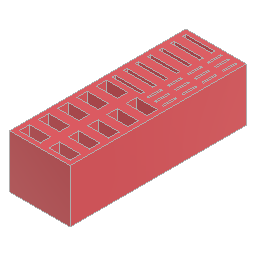
Digital-Storage-Carrier (Autodesk Fusion 360 design; units mm, degrees)
Autodesk Fusion 360 part; units mm, degrees
sketch "Sketch1 (1)" plane through (0, 0, 0) normal (0, 0, 1) x (1, 0, 0)
  line L0 (0, -297.942, 53.175) -> (51.1, -297.942, 53.175)
  line L1 (51.1, -297.942, 53.175) -> (51.1, -148.972, 53.175)
  line L2 (51.1, -148.972, 53.175) -> (0, -148.972, 53.175)
  line L3 (0, -148.972, 53.175) -> (0, -297.942, 53.175)
  line L4 (4, -285.142, 53.175) -> (21.8, -285.142, 53.175)
  line L5 (21.8, -285.142, 53.175) -> (21.8, -293.942, 53.175)
  line L6 (21.8, -293.942, 53.175) -> (4, -293.942, 53.175)
  line L7 (4, -293.942, 53.175) -> (4, -285.142, 53.175)
  line L8 (47.1, -293.942, 53.175) -> (29.3, -293.942, 53.175)
  line L9 (47.1, -285.142, 53.175) -> (47.1, -293.942, 53.175)
  line L10 (29.3, -285.142, 53.175) -> (47.1, -285.142, 53.175)
  line L11 (29.3, -293.942, 53.175) -> (29.3, -285.142, 53.175)
  line L12 (21.8, -277.642, 53.175) -> (4, -277.642, 53.175)
  line L13 (21.8, -268.842, 53.175) -> (21.8, -277.642, 53.175)
  line L14 (4, -268.842, 53.175) -> (21.8, -268.842, 53.175)
  line L15 (4, -277.642, 53.175) -> (4, -268.842, 53.175)
  line L16 (47.1, -277.642, 53.175) -> (29.3, -277.642, 53.175)
  line L17 (47.1, -268.842, 53.175) -> (47.1, -277.642, 53.175)
  line L18 (29.3, -268.842, 53.175) -> (47.1, -268.842, 53.175)
  line L19 (29.3, -277.642, 53.175) -> (29.3, -268.842, 53.175)
  line L20 (21.8, -261.342, 53.175) -> (4, -261.342, 53.175)
  line L21 (21.8, -252.542, 53.175) -> (21.8, -261.342, 53.175)
  line L22 (4, -252.542, 53.175) -> (21.8, -252.542, 53.175)
  line L23 (4, -261.342, 53.175) -> (4, -252.542, 53.175)
  line L24 (47.1, -261.342, 53.175) -> (29.3, -261.342, 53.175)
  line L25 (47.1, -252.542, 53.175) -> (47.1, -261.342, 53.175)
  line L26 (29.3, -252.542, 53.175) -> (47.1, -252.542, 53.175)
  line L27 (29.3, -261.342, 53.175) -> (29.3, -252.542, 53.175)
  line L28 (21.8, -245.042, 53.175) -> (4, -245.042, 53.175)
  line L29 (21.8, -236.242, 53.175) -> (21.8, -245.042, 53.175)
  line L30 (4, -236.242, 53.175) -> (21.8, -236.242, 53.175)
  line L31 (4, -245.042, 53.175) -> (4, -236.242, 53.175)
  line L32 (47.1, -245.042, 53.175) -> (29.3, -245.042, 53.175)
  line L33 (47.1, -236.242, 53.175) -> (47.1, -245.042, 53.175)
  line L34 (29.3, -236.242, 53.175) -> (47.1, -236.242, 53.175)
  line L35 (29.3, -245.042, 53.175) -> (29.3, -236.242, 53.175)
  line L36 (21.8, -228.742, 53.175) -> (4, -228.742, 53.175)
  line L37 (21.8, -219.942, 53.175) -> (21.8, -228.742, 53.175)
  line L38 (4, -219.942, 53.175) -> (21.8, -219.942, 53.175)
  line L39 (4, -228.742, 53.175) -> (4, -219.942, 53.175)
  line L40 (47.1, -228.742, 53.175) -> (29.3, -228.742, 53.175)
  line L41 (47.1, -219.942, 53.175) -> (47.1, -228.742, 53.175)
  line L42 (29.3, -219.942, 53.175) -> (47.1, -219.942, 53.175)
  line L43 (29.3, -228.742, 53.175) -> (29.3, -219.942, 53.175)
  line L44 (4, -212.672, 53.175) -> (28.5, -212.672, 53.175)
  line L45 (28.5, -212.672, 53.175) -> (28.5, -215.422, 53.175)
  line L46 (28.5, -215.422, 53.175) -> (4, -215.422, 53.175)
  line L47 (4, -215.422, 53.175) -> (4, -212.672, 53.175)
  line L48 (4, -202.722, 53.175) -> (28.5, -202.722, 53.175)
  line L49 (4, -205.472, 53.175) -> (4, -202.722, 53.175)
  line L50 (28.5, -205.472, 53.175) -> (4, -205.472, 53.175)
  line L51 (28.5, -202.722, 53.175) -> (28.5, -205.472, 53.175)
  line L52 (4, -192.772, 53.175) -> (28.5, -192.772, 53.175)
  line L53 (4, -195.522, 53.175) -> (4, -192.772, 53.175)
  line L54 (28.5, -195.522, 53.175) -> (4, -195.522, 53.175)
  line L55 (28.5, -192.772, 53.175) -> (28.5, -195.522, 53.175)
  line L56 (4, -182.822, 53.175) -> (28.5, -182.822, 53.175)
  line L57 (4, -185.572, 53.175) -> (4, -182.822, 53.175)
  line L58 (28.5, -185.572, 53.175) -> (4, -185.572, 53.175)
  line L59 (28.5, -182.822, 53.175) -> (28.5, -185.572, 53.175)
  line L60 (4, -172.872, 53.175) -> (28.5, -172.872, 53.175)
  line L61 (4, -175.622, 53.175) -> (4, -172.872, 53.175)
  line L62 (28.5, -175.622, 53.175) -> (4, -175.622, 53.175)
  line L63 (28.5, -172.872, 53.175) -> (28.5, -175.622, 53.175)
  line L64 (4, -162.922, 53.175) -> (28.5, -162.922, 53.175)
  line L65 (4, -165.672, 53.175) -> (4, -162.922, 53.175)
  line L66 (28.5, -165.672, 53.175) -> (4, -165.672, 53.175)
  line L67 (28.5, -162.922, 53.175) -> (28.5, -165.672, 53.175)
  line L68 (4, -152.972, 53.175) -> (28.5, -152.972, 53.175)
  line L69 (4, -155.722, 53.175) -> (4, -152.972, 53.175)
  line L70 (28.5, -155.722, 53.175) -> (4, -155.722, 53.175)
  line L71 (28.5, -152.972, 53.175) -> (28.5, -155.722, 53.175)
  line L72 (33.5, -203.692, 53.175) -> (34.8, -203.692, 53.175)
  line L73 (34.8, -203.692, 53.175) -> (34.8, -214.942, 53.175)
  line L74 (34.8, -214.942, 53.175) -> (33.5, -214.942, 53.175)
  line L75 (33.5, -214.942, 53.175) -> (33.5, -203.692, 53.175)
  line L76 (40.95, -203.692, 53.175) -> (40.95, -214.942, 53.175)
  line L77 (39.65, -203.692, 53.175) -> (40.95, -203.692, 53.175)
  line L78 (39.65, -214.942, 53.175) -> (39.65, -203.692, 53.175)
  line L79 (40.95, -214.942, 53.175) -> (39.65, -214.942, 53.175)
  line L80 (47.1, -203.692, 53.175) -> (47.1, -214.942, 53.175)
  line L81 (45.8, -203.692, 53.175) -> (47.1, -203.692, 53.175)
  line L82 (45.8, -214.942, 53.175) -> (45.8, -203.692, 53.175)
  line L83 (47.1, -214.942, 53.175) -> (45.8, -214.942, 53.175)
  line L84 (34.8, -186.782, 53.175) -> (34.8, -198.032, 53.175)
  line L85 (33.5, -186.782, 53.175) -> (34.8, -186.782, 53.175)
  line L86 (33.5, -198.032, 53.175) -> (33.5, -186.782, 53.175)
  line L87 (34.8, -198.032, 53.175) -> (33.5, -198.032, 53.175)
  line L88 (40.95, -186.782, 53.175) -> (40.95, -198.032, 53.175)
  line L89 (39.65, -186.782, 53.175) -> (40.95, -186.782, 53.175)
  line L90 (39.65, -198.032, 53.175) -> (39.65, -186.782, 53.175)
  line L91 (40.95, -198.032, 53.175) -> (39.65, -198.032, 53.175)
  line L92 (47.1, -186.782, 53.175) -> (47.1, -198.032, 53.175)
  line L93 (45.8, -186.782, 53.175) -> (47.1, -186.782, 53.175)
  line L94 (45.8, -198.032, 53.175) -> (45.8, -186.782, 53.175)
  line L95 (47.1, -198.032, 53.175) -> (45.8, -198.032, 53.175)
  line L96 (34.8, -169.872, 53.175) -> (34.8, -181.122, 53.175)
  line L97 (33.5, -169.872, 53.175) -> (34.8, -169.872, 53.175)
  line L98 (33.5, -181.122, 53.175) -> (33.5, -169.872, 53.175)
  line L99 (34.8, -181.122, 53.175) -> (33.5, -181.122, 53.175)
  line L100 (40.95, -169.872, 53.175) -> (40.95, -181.122, 53.175)
  line L101 (39.65, -169.872, 53.175) -> (40.95, -169.872, 53.175)
  line L102 (39.65, -181.122, 53.175) -> (39.65, -169.872, 53.175)
  line L103 (40.95, -181.122, 53.175) -> (39.65, -181.122, 53.175)
  line L104 (47.1, -169.872, 53.175) -> (47.1, -181.122, 53.175)
  line L105 (45.8, -169.872, 53.175) -> (47.1, -169.872, 53.175)
  line L106 (45.8, -181.122, 53.175) -> (45.8, -169.872, 53.175)
  line L107 (47.1, -181.122, 53.175) -> (45.8, -181.122, 53.175)
  line L108 (34.8, -152.962, 53.175) -> (34.8, -164.212, 53.175)
  line L109 (33.5, -152.962, 53.175) -> (34.8, -152.962, 53.175)
  line L110 (33.5, -164.212, 53.175) -> (33.5, -152.962, 53.175)
  line L111 (34.8, -164.212, 53.175) -> (33.5, -164.212, 53.175)
  line L112 (40.95, -152.962, 53.175) -> (40.95, -164.212, 53.175)
  line L113 (39.65, -152.962, 53.175) -> (40.95, -152.962, 53.175)
  line L114 (39.65, -164.212, 53.175) -> (39.65, -152.962, 53.175)
  line L115 (40.95, -164.212, 53.175) -> (39.65, -164.212, 53.175)
  line L116 (47.1, -152.962, 53.175) -> (47.1, -164.212, 53.175)
  line L117 (45.8, -152.962, 53.175) -> (47.1, -152.962, 53.175)
  line L118 (45.8, -164.212, 53.175) -> (45.8, -152.962, 53.175)
  line L119 (47.1, -164.212, 53.175) -> (45.8, -164.212, 53.175)
  point P0 (0, -595.884)
sketch "Sketch1" plane through (0, 0, 3.175) normal (0, 0, 1) x (-1, 0, 0)
  line L0 (0, 0) -> (0, 297.942)
  line L1 (0, 297.942) -> (-407.924, 297.942)
  line L2 (-407.924, 297.942) -> (-407.924, 0)
  line L3 (-407.924, 0) -> (0, 0)
  line L4 (0, 297.942) -> (-51.1, 297.942)
  line L5 (-51.1, 297.942) -> (-51.1, 148.972)
  line L6 (-51.1, 148.972) -> (0, 148.972)
  line L7 (0, 148.972) -> (0, 297.942)
  dimension "d1" = 51.1
  dimension "d2" = 148.97
  constraint horizontal L4
  constraint vertical L5
  constraint horizontal L6
  constraint vertical L7
  constraint coincident L0.end L1.start
  measures "d1" distance of L0.end L4.end
  measures "d2" distance of L0.end L6.end
extrude "Extrude1" add sketch "Sketch1" along normal blind 45 contours L0 L1 L4 L5 L6 L7
extrude "Extrude2" cut sketch "Sketch1 (1)" against normal blind 37.5 contours L4 L5 L6 L7 | L8 L9 L10 L11 | L12 L13 L14 L15 | L16 L17 L18 L19 | L20 L21 L22 L23 | L24 L25 L26 L27 | L28 L29 L30 L31 | L32 L33 L34 L35 | L36 L37 L38 L39 | L40 L41 L42 L43 in plane through (0, 0, 53.175) normal (0, 0, 1)
extrude "Extrude3" cut sketch "Sketch1 (1)" against normal blind 21 contours L44 L45 L46 L47 | L48 L49 L50 L51 | L52 L53 L54 L55 | L56 L57 L58 L59 | L60 L61 L62 L63 | L64 L65 L66 L67 | L68 L69 L70 L71 in plane through (0, 0, 53.175) normal (0, 0, 1)
extrude "Extrude4" cut sketch "Sketch1 (1)" against normal blind 9.5 contours L72 L73 L74 L75 | L76 L77 L78 L79 | L80 L81 L82 L83 | L84 L85 L86 L87 | L88 L89 L90 L91 | L92 L93 L94 L95 | L96 L97 L98 L99 | L100 L101 L102 L103 | L104 L105 L106 L107 | L108 L109 L110 L111 | L112 L113 L114 L115 | L116 L117 L118 L119 in plane through (0, 0, 53.175) normal (0, 0, 1)
equation "d1 = DigitalStorageWidth"
equation "d2 = DigitalStorageLength"
equation "d3 = DigitalStorageDepth"
equation "DigitalStorageLength = 148.97 mm"
equation "DigitalStorageWidth = 51.1 mm"
equation "DigitalStorageDepth = 45 mm"
